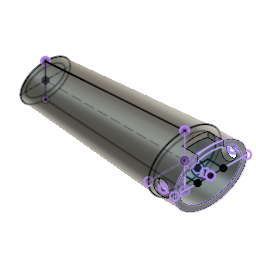
Forearm (Autodesk Fusion 360 design; units mm, degrees)
Autodesk Fusion 360 part; units mm, degrees
sketch "ForearmProfile" plane through (0, 0, 0) normal (0, 1, 0) x (1, 0, 0)
  line L0 (0, 0) -> (0, -100)
  line L1 (0, -50) -> (-270, -50) construction
  line L2 (-270, -50) -> (-270, -82) construction
  line L3 (-270, -82) -> (-270, -18)
  line L4 (-270, -82) -> (0, -100)
  line L5 (-270, -18) -> (0, 0)
  dimension "d1" = 270
  dimension "d2" = 100
  dimension "d3" = 32
  dimension "d4" = 64
  constraint coincident L0.start L5.end
  constraint vertical L0
  constraint horizontal L1
  constraint midpoint L0 L1.start
  constraint perpendicular L1 L2
  constraint parallel L2 L3
  measures "d1" distance of L1.start L1.end
  measures "d2" distance of L0.start L0.end
  measures "d3" distance of L1.end L2.end
  measures "d4" distance of L2.end L3.end
sketch "EndOfForearmProfile" plane through (0, 0, 0) normal (1, 0, 0) x (0, 1, 0)
  line L0 (0, 0) -> (0, 100)
  ellipse E0 centre (0, 50) end of major axis (70, 50) minor radius 50
  line L1 (-70, 50) -> (70, 50)
  line L2 (0, 0) -> (0, 100)
  ellipse E1 centre (0, 50) end of major axis (60, 50) minor radius 40
  line L3 (-60, 50) -> (60, 50)
  line L4 (0, 10) -> (0, 90)
  dimension "d5" = 140
  dimension "d8" = 10
  dimension "d9" = 10
  constraint midpoint L0 E0.centre
  constraint perpendicular L0 L1
  constraint coincident E0 L1.start
  constraint coincident E0 L1.end
  constraint coincident L0.start E0
  constraint concentric E0 E1
  constraint perpendicular L0 L3
  constraint coincident E1 L3.start
  constraint coincident E1 L3.end
  constraint coincident E1 L4.start
  constraint coincident E1 L4.end
  measures "d5" distance of E0
  measures "d8" distance of L0.end L4.end
  measures "d9" distance of L1.end L3.end
ref_plane "WorkPlane1" through (-270, 35, 50) normal (1, 0, 0) x (0, 1, 0)
sketch "DistalForarmProfile" plane through (-270, 37.5, 50) normal (1, 0, 0) x (0, 1, 0)
  line L0 (-37.5, 32) -> (-37.5, -32)
  ellipse E0 centre (-37.5, 0) end of major axis (-85.5, 0) minor radius 32
  line L1 (10.5, 0) -> (-85.5, 0)
  line L2 (-37.5, 32) -> (-37.5, -32)
  ellipse E1 centre (-37.5, 0) end of major axis (-75.5, 0) minor radius 22
  line L3 (0.5, 0) -> (-75.5, 0)
  line L4 (-37.5, 22) -> (-37.5, -22)
  point P0 (-37.5, 32)
  dimension "d7" = 96
  dimension "d10" = 10
  dimension "d11" = 10
  constraint midpoint L0 E0.centre
  constraint perpendicular L0 L1
  constraint coincident E0 L1.start
  constraint coincident E0 L1.end
  constraint coincident L0.end E0
  constraint concentric E0 E1
  constraint perpendicular L0 L3
  constraint coincident E1 L3.start
  constraint coincident E1 L3.end
  constraint coincident E1 L4.start
  constraint coincident E1 L4.end
  measures "d7" distance of E0
  measures "d10" distance of L4.start P0
  measures "d11" distance of L1.end L3.end
form "Form1" [no effect]
loft "Loft1" add profiles "EndOfForearmProfile", "DistalForarmProfile" section 1 contours L0 E0 L1 L2 E1 | L0 E0 L1 L2 E1 picked at (16.881, 5.0389) picked at (22.7654, 93.7465) section 2 contours L0 E0 L1 L2 E1 | L0 E0 L1 L2 E1 picked at (-23.402, 27.1386) picked at (-34.4801, -28.4749)
loft "Loft2" add profiles "EndOfForearmProfile", "DistalForarmProfile" section 1 contours L0 E0 L1 L2 E1 | L0 E0 L1 L2 E1 picked at (-22.7654, 6.2535) picked at (-16.881, 94.9611) section 2 contours L0 E0 L1 L2 E1 | L0 E0 L1 L2 E1 picked at (-40.5199, 28.4749) picked at (-51.598, -27.1386)
sketch "LenghtOfConnection" plane through (0, 0, 0) normal (0, 1, 0) x (1, 0, 0)
  line L0 (0, -50) -> (50, -50)
  line L1 (0, 0) -> (0, -100)
  line L2 (0, 0) -> (0, -100)
  dimension "d12" = 50
  constraint horizontal L0
  constraint midpoint L0.start L2
  measures "d12" distance of L0.start L0.end
ref_plane "WorkPlane2" through (50, 35, 50) normal (1, 0, 0) x (0, 1, 0)
sketch "MedialElbow" plane through (50, 37.5, 50) normal (1, 0, 0) x (0, 1, 0)
  ellipse E0 centre (-37.5, 0) end of major axis (32.5, 0) minor radius 50
  ellipse E1 centre (-37.5, 0) end of major axis (22.5, 0) minor radius 40
loft "Loft3" add profiles "MedialElbow", "EndOfForearmProfile" section 1 section 2 contours L0 E0 L1 L2 E1 | L0 E0 L1 L2 E1 | L0 E0 L1 L2 E1 | L0 E0 L1 L2 E1
extrude "Extrude1" cut sketch "MedialElbow" against normal blind 50 contours E1
sketch "Holes?" plane through (0, 0, 0) normal (0, 1, 0) x (1, 0, 0)
  line L0 (0, -50) -> (50, -50)
  circle A0 centre (25, -50) radius 15
  dimension "d16" = 30
  constraint midpoint L0 A0.centre
  measures "d16" diameter of A0
extrude "Extrude2" cut sketch "Holes?" along normal through all and the other way through all
sketch "Joints" plane through (0, 0, 0) normal (0, 1, 0) x (1, 0, 0)
  circle A0 centre (25, -50) radius 15
ref_plane "WorkPlane5" through (0, 0, 50) normal (0, 0, 1) x (1, 0, 0)
sketch "Clearance" plane through (0, 0, 50) normal (0, 0, 1) x (1, 0, 0)
  spline S0 degree 3 poles (27.9111, 66.9) (27.9111, 66.9) (28.8849, 66.9831) (29.8496, 67.1078) (32.6156, 67.573) (34.287, 68.0058) (36.9254, 68.8077) (38.0763, 69.232) (39.2297, 69.6821) (39.5223, 69.8018) (39.9076, 69.9608) (40, 70) (40, 70) (39.9076, 69.9608) (39.5223, 69.8018) (39.2297, 69.6821) (38.0763, 69.232) (36.9254, 68.8077) (34.287, 68.0058) (32.6156, 67.573) (29.8496, 67.1078) (28.8849, 66.9831) (26.9373, 66.8169) (25.9544, 66.7757) (25, 66.7757) knots 0 0.286317 0.286317 0.286317 0.286317 0.572633 0.572633 1.145266 1.145266 1.717567 1.717567 2.003718 2.003718 2.289868 2.289868 2.576019 2.576019 2.862169 2.862169 3.43447 3.43447 4.007103 4.007103 4.29342 4.29342 4.579737 4.579737 4.579737 4.579737
  spline S1 degree 3 poles (27.9111, -66.9) (27.9111, -66.9) (28.8849, -66.9831) (29.8496, -67.1078) (32.6156, -67.573) (34.287, -68.0058) (36.9254, -68.8077) (38.0763, -69.232) (39.2297, -69.6821) (39.5223, -69.8018) (39.9076, -69.9608) (40, -70) (40, -70) (39.9076, -69.9608) (39.5223, -69.8018) (39.2297, -69.6821) (38.0763, -69.232) (36.9254, -68.8077) (34.287, -68.0058) (32.6156, -67.573) (29.8496, -67.1078) (28.8849, -66.9831) (26.9373, -66.8169) (25.9544, -66.7757) (25, -66.7757) knots 4.579737 4.866053 4.866053 4.866053 4.866053 5.15237 5.15237 5.725003 5.725003 6.297304 6.297304 6.583454 6.583454 6.869605 6.869605 7.155755 7.155755 7.441906 7.441906 8.014207 8.014207 8.58684 8.58684 8.873157 8.873157 9.159473 9.159473 9.159473 9.159473
  line L0 (50, 70) -> (50, -70)
  line L1 (0, 0) -> (0, 70)
  line L2 (0, -70) -> (0, 0)
  line L3 (40, 0) -> (10, 0)
  line L4 (50, -25) -> (50, 25)
  line L5 (50, 25) -> (20, 25)
  line L6 (20, 25) -> (20, -25)
  line L7 (20, -25) -> (50, -25)
  dimension "d25" = 30
  dimension "d26" = 50
  constraint perpendicular L4 L5
  constraint parallel L4 L6
  constraint parallel L5 L7
  constraint coincident L0 L4.end
  constraint coincident L0 L4.start
  constraint midpoint L0 L4
  measures "d25" distance of L4 L6
  measures "d26" distance of L4.start L4.end
extrude "Extrude3" cut sketch "Clearance" along normal through all
ref_plane "WorkPlane4" through (0, 0, 50) normal (0, 0, 1) x (1, 0, 0)
equation "d3 = ( d2 / 2.5 ) * 0.8"
equation "d4 = d3 * 2"
equation "d5 = d2 * 1.4"
equation "d6 = -d1"
equation "d7 = d4 * 1.5"
equation "d13 = d12"
equation "d14 = -d12"
named bodies: "Forearm"
